Autodesk Inventor part; units mm, degrees
note: some values were not read from the file. Chosen so that the rebuilt part matches the saved one: direction of "Hole2".
(part 12 of 20)
  line L725 (-87.264021, -27.045907) -> (-87.291941, -27.048237)
  line L726 (-87.250271, -24.95924) -> (-87.458208, -24.976595)
  line L727 (-87.288621, -27.057017) -> (-87.239208, -27.052892)
  ellipse E573 centre (-87.05098, -26.778416) end of major axis (-86.983232, -26.537771) minor radius 0.214215 (-87.262006, -26.740129) -> (-87.262743, -26.851991) ccw
  ellipse E574 centre (-87.040523, -25.191443) end of major axis (-86.972774, -24.950798) minor radius 0.214215 (-87.251549, -25.153156) -> (-87.252286, -25.265018) ccw
  spline S72 degree 3 poles (-86.844242, -26.766257) (-86.846137, -26.752647) (-86.849873, -26.725818) (-86.862228, -26.68763) (-86.878945, -26.652628) (-86.900084, -26.621606) (-86.92513, -26.595311) (-86.953734, -26.574537) (-86.980247, -26.56254) (-87.002525, -26.556638) (-87.019846, -26.554098) (-87.037692, -26.553557) (-87.056005, -26.555112) (-87.074575, -26.558831) (-87.093006, -26.564642) (-87.110888, -26.572422) (-87.133717, -26.5852) (-87.16009, -26.605396) (-87.187412, -26.63502) (-87.209849, -26.669164) (-87.227399, -26.706727) (-87.23392, -26.733619) (-87.237193, -26.747114) knots 0 0 0 0 0.06705351 0.13217076 0.19521445 0.25608707 0.314845 0.37183317 0.42783149 0.45589727 0.48426542 0.51319288 0.54296576 0.57389196 0.60556318 0.63723227 0.66902668 0.73324746 0.79861392 0.865047 0.93227307 1 1 1 1
  spline S73 degree 3 poles (-87.262006, -26.740129) (-87.260244, -26.733331) (-87.256712, -26.719711) (-87.246016, -26.693462) (-87.227942, -26.662404) (-87.199749, -26.629194) (-87.166328, -26.600489) (-87.128819, -26.577002) (-87.088383, -26.559452) (-87.046165, -26.548593) (-87.010271, -26.545789) (-86.981977, -26.547757) (-86.961175, -26.551403) (-86.941138, -26.55724) (-86.922223, -26.565108) (-86.90469, -26.574815) (-86.883243, -26.589954) (-86.859658, -26.612961) (-86.836903, -26.6456) (-86.819582, -26.682128) (-86.807069, -26.721446) (-86.802924, -26.748832) (-86.800834, -26.762634) knots 0 0 0 0 0.03133748 0.06278121 0.12629735 0.19093644 0.25645898 0.32231967 0.3878749 0.45257734 0.51618281 0.54767829 0.57907039 0.61032535 0.64070557 0.67038635 0.69964994 0.75776174 0.81647804 0.87644136 0.93772561 1 1 1 1
  spline S74 degree 3 poles (-86.801575, -26.874947) (-86.803934, -26.887405) (-86.808531, -26.911671) (-86.823414, -26.945046) (-86.84347, -26.974042) (-86.868727, -26.998205) (-86.898529, -27.017194) (-86.932394, -27.030679) (-86.969811, -27.038356) (-87.010303, -27.03992) (-87.052914, -27.035123) (-87.095691, -27.024267) (-87.136319, -27.007228) (-87.173004, -26.984845) (-87.204936, -26.957641) (-87.227026, -26.931239) (-87.241417, -26.90832) (-87.250446, -26.890314) (-87.257822, -26.871543) (-87.2611, -26.858518) (-87.262743, -26.851991) knots 0 0 0 0 0.06022667 0.11730293 0.17254203 0.22724068 0.28263107 0.33984452 0.39989686 0.46369518 0.53205848 0.6034638 0.67318901 0.7411164 0.8073508 0.87214279 0.90417982 0.93607992 0.96796844 1 1 1 1
  spline S75 degree 3 poles (-87.23793, -26.858977) (-87.237265, -26.862275) (-87.23594, -26.868848) (-87.233332, -26.878531) (-87.230299, -26.888022) (-87.225663, -26.900374) (-87.218799, -26.91531) (-87.20898, -26.932343) (-87.197734, -26.948418) (-87.185176, -26.963452) (-87.171525, -26.9775) (-87.161568, -26.98592) (-87.156591, -26.990129) knots 0 0 0 0 0.06406043 0.12763921 0.19082759 0.25370622 0.37876994 0.50330734 0.62760512 0.75181377 0.87596664 1 1 1 1
  spline S76 degree 3 poles (-86.94314, -27.035596) (-86.939586, -27.03406) (-86.932537, -27.031015) (-86.922574, -27.025353) (-86.913208, -27.018983) (-86.904463, -27.011852) (-86.896326, -27.004009) (-86.888792, -26.995478) (-86.881851, -26.986289) (-86.875498, -26.976469) (-86.869724, -26.966046) (-86.864521, -26.955048) (-86.859882, -26.9435) (-86.855799, -26.931431) (-86.852262, -26.918867) (-86.849276, -26.905834) (-86.846786, -26.892364) (-86.845588, -26.883204) (-86.844982, -26.87857) knots 0 0 0 0 0.05963345 0.11825449 0.17626219 0.23403402 0.29191894 0.35023204 0.40925111 0.46921525 0.53032509 0.59274441 0.65660269 0.7219981 0.78900076 0.85765603 0.92798753 1 1 1 1
  spline S77 degree 3 poles (-86.833785, -25.179284) (-86.83568, -25.165674) (-86.839416, -25.138845) (-86.851771, -25.100657) (-86.868488, -25.065655) (-86.889626, -25.034633) (-86.914673, -25.008338) (-86.943277, -24.987564) (-86.969789, -24.975567) (-86.992068, -24.969665) (-87.009388, -24.967125) (-87.027235, -24.966584) (-87.045548, -24.968139) (-87.064118, -24.971858) (-87.082548, -24.977669) (-87.10043, -24.985449) (-87.12326, -24.998227) (-87.149633, -25.018423) (-87.176955, -25.048047) (-87.199392, -25.082191) (-87.216942, -25.119754) (-87.223463, -25.146646) (-87.226736, -25.160141) knots 0 0 0 0 0.06705351 0.13217076 0.19521445 0.25608707 0.314845 0.37183317 0.42783149 0.45589727 0.48426542 0.51319288 0.54296576 0.57389196 0.60556318 0.63723227 0.66902668 0.73324746 0.79861392 0.865047 0.93227307 1 1 1 1
  spline S78 degree 3 poles (-87.251549, -25.153156) (-87.249786, -25.146357) (-87.246255, -25.132738) (-87.235559, -25.106489) (-87.217485, -25.075431) (-87.189292, -25.042221) (-87.155871, -25.013516) (-87.118362, -24.990029) (-87.077926, -24.972479) (-87.035708, -24.96162) (-86.999814, -24.958816) (-86.97152, -24.960784) (-86.950718, -24.96443) (-86.930681, -24.970267) (-86.911765, -24.978135) (-86.894233, -24.987842) (-86.872786, -25.002981) (-86.849201, -25.025988) (-86.826446, -25.058627) (-86.809125, -25.095155) (-86.796612, -25.134473) (-86.792467, -25.161859) (-86.790377, -25.175661) knots 0 0 0 0 0.03133748 0.06278121 0.12629735 0.19093644 0.25645898 0.32231967 0.3878749 0.45257734 0.51618281 0.54767829 0.57907039 0.61032535 0.64070557 0.67038635 0.69964994 0.75776174 0.81647804 0.87644136 0.93772561 1 1 1 1
  spline S79 degree 3 poles (-86.791117, -25.287974) (-86.793477, -25.300432) (-86.798074, -25.324698) (-86.812957, -25.358073) (-86.833013, -25.387069) (-86.85827, -25.411232) (-86.888072, -25.430221) (-86.921937, -25.443706) (-86.959354, -25.451383) (-86.999846, -25.452947) (-87.042457, -25.44815) (-87.085233, -25.437294) (-87.125862, -25.420255) (-87.162546, -25.397872) (-87.194479, -25.370668) (-87.216569, -25.344266) (-87.23096, -25.321347) (-87.239988, -25.303341) (-87.247365, -25.28457) (-87.250643, -25.271545) (-87.252286, -25.265018) knots 0 0 0 0 0.06022667 0.11730293 0.17254203 0.22724068 0.28263107 0.33984452 0.39989686 0.46369518 0.53205848 0.6034638 0.67318901 0.7411164 0.8073508 0.87214279 0.90417982 0.93607992 0.96796844 1 1 1 1
  spline S80 degree 3 poles (-87.227473, -25.272004) (-87.226808, -25.275302) (-87.225483, -25.281875) (-87.222875, -25.291558) (-87.219842, -25.301049) (-87.215205, -25.3134) (-87.208342, -25.328337) (-87.198522, -25.34537) (-87.187277, -25.361445) (-87.174719, -25.376479) (-87.161068, -25.390527) (-87.151111, -25.398947) (-87.146134, -25.403156) knots 0 0 0 0 0.06406043 0.12763921 0.19082759 0.25370622 0.37876994 0.50330734 0.62760512 0.75181377 0.87596664 1 1 1 1
  spline S81 degree 3 poles (-86.932683, -25.448623) (-86.929129, -25.447087) (-86.92208, -25.444042) (-86.912117, -25.43838) (-86.90275, -25.43201) (-86.894006, -25.424879) (-86.885869, -25.417036) (-86.878334, -25.408505) (-86.871394, -25.399316) (-86.865041, -25.389496) (-86.859267, -25.379073) (-86.854064, -25.368074) (-86.849424, -25.356527) (-86.845342, -25.344458) (-86.841805, -25.331894) (-86.838819, -25.318861) (-86.836329, -25.305391) (-86.835131, -25.296231) (-86.834525, -25.291597) knots 0 0 0 0 0.05963345 0.11825449 0.17626219 0.23403402 0.29191894 0.35023204 0.40925111 0.46921525 0.53032509 0.59274441 0.65660269 0.7219981 0.78900076 0.85765603 0.92798753 1 1 1 1
  ellipse E575 centre (-86.922017, -26.784779) end of major axis (-86.901223, -27.033912) minor radius 0.122746 (-86.801575, -26.874947) -> (-86.800834, -26.762634) ccw
  ellipse E576 centre (-86.965424, -26.788402) end of major axis (-86.986218, -26.539268) minor radius 0.122746 (-86.844982, -26.87857) -> (-86.844242, -26.766257) ccw
  ellipse E577 centre (-86.91156, -25.197806) end of major axis (-86.890766, -25.446939) minor radius 0.122746 (-86.791117, -25.287974) -> (-86.790377, -25.175661) ccw
  ellipse E578 centre (-86.954967, -25.201429) end of major axis (-86.975761, -24.952295) minor radius 0.122746 (-86.834525, -25.291597) -> (-86.833785, -25.179284) ccw
  ellipse E579 centre (-87.026167, -26.785401) end of major axis (-87.093915, -27.026047) minor radius 0.214215 (-87.237193, -26.747114) -> (-87.23793, -26.858977) ccw
  ellipse E580 centre (-87.01571, -25.198428) end of major axis (-87.083458, -25.439074) minor radius 0.214215 (-87.226736, -25.160141) -> (-87.227473, -25.272004) ccw
  ellipse E581 centre (-87.096286, -27.093129) end of major axis (-86.808292, -27.095027) minor radius 0.045287 (-86.846258, -27.072261) -> (-87.239208, -27.052892) ccw
  ellipse E582 centre (-87.096286, -27.093129) end of major axis (-87.434279, -27.090902) minor radius 0.05315 (-86.802851, -27.068638) -> (-87.264021, -27.045907) ccw
  ellipse E583 centre (-87.082536, -25.006462) end of major axis (-87.420529, -25.004235) minor radius 0.05315 (-86.789101, -24.981971) -> (-87.250271, -24.95924) ccw
  line L728 (-86.643643, -27.113459) -> (-86.802851, -27.068638)
  line L729 (-86.789101, -24.981971) -> (-86.772465, -24.986654)
  line L730 (-86.756765, -24.991074) -> (-86.743873, -24.994703)
  line L731 (-86.685676, -27.117469) -> (-86.846258, -27.072261)
  line L732 (-107.562177, -25.014438) -> (-107.45568, -25.019413)
  ellipse E584 centre (-86.54231, -24.68723) end of major axis (-86.626787, -24.985498) minor radius 0.255849 (-86.550009, -24.992758) -> (-86.536151, -24.991163) ccw
  line L733 (-86.536151, -24.991163) -> (-86.46886, -25.010221)
  line L734 (-86.599622, -24.996924) -> (-86.550009, -24.992758)
  arc A8 (-108.822768, -25.15652) -> (-108.721613, -25.266481) centre (-108.550766, -25.007808) ccw
  ellipse E585 centre (-86.547255, -25.103114) end of major axis (-86.105319, -25.125457) minor radius 0.079087 (-86.348028, -25.04218) -> (-86.360093, -25.040539) ccw
  arc A9 (-85.268509, -25.261265) -> (-85.143186, -25.138916) centre (-85.413584, -24.987307) ccw
  ellipse E586 centre (-107.271615, -24.666993) end of major axis (-107.176326, -24.961985) minor radius 0.274042 (-107.284377, -24.971637) -> (-107.269597, -24.97313) ccw
  line L735 (-107.299761, -24.976606) -> (-107.284377, -24.971637)
  line L736 (-107.269597, -24.97313) -> (-107.130091, -24.98313)
  ellipse E587 centre (-87.344737, -24.633834) end of major axis (-87.318953, -24.94276) minor radius 0.152204 (-87.355436, -24.937038) -> (-87.346755, -24.939971) ccw
  line L737 (-87.455183, -24.945363) -> (-87.355436, -24.937038)
  ellipse E588 centre (-86.781051, -24.661503) end of major axis (-86.865059, -24.959903) minor radius 0.265627 (-86.783068, -24.967639) -> (-86.768741, -24.96601) ccw
  line L738 (-86.768741, -24.96601) -> (-86.718934, -24.980032)
  line L739 (-86.834568, -24.971938) -> (-86.783068, -24.967639)
  line L740 (-87.346755, -24.939971) -> (-87.294003, -24.954822)
  ellipse E589 centre (-87.203964, -25.032925) end of major axis (-86.761473, -25.035841) minor radius 0.069582 (-86.983801, -24.97398) -> (-87.009912, -24.971636) ccw
  arc A10 (-107.361771, -27.097474) -> (-107.495936, -27.121179) centre (-107.376234, -27.407136) ccw
  line L741 (-107.495936, -27.121179) -> (-107.541681, -27.140328)
  line L742 (-107.035954, -27.112691) -> (-107.361771, -27.097474)
  arc A11 (-107.768298, -27.148427) -> (-107.783494, -27.154591) centre (-107.659411, -27.438674) ccw
  arc A12 (-107.648929, -27.128852) -> (-107.740372, -27.139433) centre (-107.659411, -27.438674) ccw
  line L743 (-107.783494, -27.154591) -> (-107.873673, -27.193979)
  line L744 (-107.524335, -27.133067) -> (-107.648929, -27.128852)
  arc A13 (-106.402931, -32.497897) -> (-106.400859, -32.497157) centre (-106.805429, -31.367412) ccw
  line L745 (-87.818851, -31.56199) -> (-87.720015, -32.505823)
  line L746 (-106.184231, -31.56199) -> (-106.283067, -32.505823)
  arc A14 (-87.602223, -32.497157) -> (-87.600151, -32.497897) centre (-87.197653, -31.367412) ccw
  arc A15 (-90.598492, -35.33817) -> (-90.48289, -35.312603) centre (-90.799519, -34.155129) ccw
  line L747 (-90.29603, -34.046814) -> (-90.28314, -34.105092)
  arc A16 (-103.520192, -35.312603) -> (-103.40459, -35.33817) centre (-103.203563, -34.155129) ccw
  line L748 (-103.707052, -34.046814) -> (-103.719942, -34.105092)
  arc A17 (-107.267726, -34.321251) -> (-106.77775, -34.355522) centre (-106.940784, -33.166648) ccw
  line L749 (-108.036328, -21.696665) -> (-108.026854, -21.884052)
  line L750 (-107.975177, -22.906217) -> (-107.96796, -23.048964)
  line L751 (-107.657328, -29.193171) -> (-107.540315, -31.507663)
  line L752 (-107.48592, -32.583586) -> (-107.451463, -33.265126)
  arc A18 (-104.353756, -35.223246) -> (-104.235408, -35.229466) centre (-104.231678, -34.029472) ccw
  line L753 (-103.716719, -34.043774) -> (-103.719942, -34.105092)
  line L754 (-104.706079, -33.243459) -> (-104.756348, -34.199934)
  line L755 (-91.493695, -33.096855) -> (-91.477416, -33.173659)
  arc A19 (-88.109461, -35.54276) -> (-87.810531, -35.509047) centre (-88.093417, -34.342867) ccw
  line L756 (-87.667, -33.528456) -> (-87.560911, -34.469138)
  line L757 (-88.69143, -33.635739) -> (-88.584423, -34.584568)
  arc A20 (-106.192551, -35.509047) -> (-105.893621, -35.54276) centre (-105.909665, -34.342867) ccw
  line L758 (-105.311652, -33.635739) -> (-105.418659, -34.584568)
  line L759 (-106.336082, -33.528456) -> (-106.442171, -34.469138)
  line L760 (-102.509387, -33.096855) -> (-102.525666, -33.173659)
  arc A21 (-89.767674, -35.229466) -> (-89.649326, -35.223246) centre (-89.771404, -34.029472) ccw
  line L761 (-89.297003, -33.243459) -> (-89.246734, -34.199934)
  line L762 (-90.286363, -34.043774) -> (-90.28314, -34.105092)
  arc A22 (-87.225332, -34.355522) -> (-86.735356, -34.321251) centre (-87.062298, -33.166648) ccw
  line L763 (-85.966754, -21.696665) -> (-85.976228, -21.884052)
  line L764 (-86.027905, -22.906217) -> (-86.033482, -23.016517)
  line L765 (-86.344197, -29.162376) -> (-86.462767, -31.507663)
  line L766 (-86.517162, -32.583586) -> (-86.551619, -33.265126)
  line L767 (-106.187707, -21.753853) -> (-106.187436, -21.794963)
  line L768 (-106.139211, -29.113475) -> (-106.135988, -29.602592)
  line L769 (-88.008683, -28.994618) -> (-87.858681, -30.530102)
  line L770 (-105.994399, -28.994618) -> (-106.144401, -30.530102)
  line L771 (-87.815376, -21.753853) -> (-87.815646, -21.794963)
  line L772 (-87.863801, -29.102841) -> (-87.867094, -29.602592)
  ellipse E590 centre (-107.19283, -15.992439) end of major axis (-108.892291, -16.03526) minor radius 0.28459 (-108.378765, -15.817576) -> (-108.892291, -16.03526) ccw
  line L773 (-108.888419, -16.188929) -> (-108.892291, -16.03526)
  ellipse E591 centre (-86.810252, -15.992439) end of major axis (-85.110791, -16.03526) minor radius 0.28459 (-85.110791, -16.03526) -> (-85.624317, -15.817576) ccw
  line L774 (-85.114663, -16.188929) -> (-85.110791, -16.03526)
  ellipse E592 centre (-107.715782, -17.837411) end of major axis (-109.413614, -17.923248) minor radius 0.303839 (-108.663788, -17.631425) -> (-109.413614, -17.923248) ccw
  line L775 (-109.406367, -18.066578) -> (-109.413614, -17.923248)
  ellipse E593 centre (-86.2873, -17.837411) end of major axis (-84.589468, -17.923248) minor radius 0.303839 (-84.589468, -17.923248) -> (-85.339294, -17.631425) ccw
  line L776 (-84.596715, -18.066578) -> (-84.589468, -17.923248)
  ellipse E594 centre (-89.901015, -14.920785) end of major axis (-88.209069, -14.755498) minor radius 0.097712 (-88.209069, -14.755498) -> (-88.726459, -14.735759) ccw
  line L777 (-88.184691, -15.005043) -> (-88.209069, -14.755498)
  ellipse E595 centre (-104.102067, -14.920785) end of major axis (-105.794013, -14.755498) minor radius 0.097712 (-105.276623, -14.735759) -> (-105.794013, -14.755498) ccw
  line L778 (-105.818391, -15.005043) -> (-105.794013, -14.755498)
  ellipse E596 centre (-107.115847, -19.047722) end of major axis (-105.616323, -19.009938) minor radius 0.251109 (-106.242723, -18.822124) -> (-106.866306, -18.793926) ccw
  ellipse E597 centre (-107.115847, -19.047722) end of major axis (-105.21645, -18.999863) minor radius 0.318071 (-106.234573, -18.744288) -> (-108.180062, -18.810245) ccw
  ellipse E598 centre (-107.18538, -16.288111) end of major axis (-109.084778, -16.33597) minor radius 0.318071 (-107.887293, -16.009653) -> (-109.084778, -16.33597) ccw
  line L779 (-109.050041, -17.714567) -> (-109.084778, -16.33597)
  ellipse E599 centre (-89.550588, -19.969597) end of major axis (-87.66092, -19.771717) minor radius 0.08119 (-87.819088, -19.82131) -> (-87.877602, -19.756773) ccw
  ellipse E600 centre (-89.841934, -17.187367) end of major axis (-87.952267, -16.989487) minor radius 0.08119 (-88.062989, -16.97389) -> (-88.463494, -16.987448) ccw
  line L780 (-87.66092, -19.771717) -> (-87.86609, -17.812439)
  ellipse E601 centre (-104.452494, -19.969597) end of major axis (-106.342162, -19.771717) minor radius 0.08119 (-106.12548, -19.756773) -> (-106.183994, -19.82131) ccw
  ellipse E602 centre (-104.161148, -17.187367) end of major axis (-106.050815, -16.989487) minor radius 0.08119 (-105.539588, -16.987448) -> (-105.940093, -16.97389) ccw
  line L781 (-106.342162, -19.771717) -> (-106.136992, -17.812439)
  ellipse E603 centre (-86.887235, -19.047722) end of major axis (-85.387711, -19.085505) minor radius 0.251109 (-87.136776, -18.793926) -> (-87.760359, -18.822124) ccw
  ellipse E604 centre (-86.887235, -19.047722) end of major axis (-84.987838, -19.095581) minor radius 0.318071 (-85.82302, -18.810245) -> (-87.768509, -18.744288) ccw
  ellipse E605 centre (-86.817702, -16.288111) end of major axis (-84.918305, -16.33597) minor radius 0.318071 (-84.918305, -16.33597) -> (-86.115789, -16.009653) ccw
  line L782 (-84.953041, -17.714567) -> (-84.918305, -16.33597)
  ellipse E606 centre (-107.561776, -20.883606) end of major axis (-109.059863, -20.959344) minor radius 0.268093 (-106.281023, -20.681668) -> (-108.752123, -21.104847) ccw
  ellipse E607 centre (-107.561776, -20.883606) end of major axis (-109.459353, -20.979541) minor radius 0.339584 (-106.268597, -20.571487) -> (-108.746952, -21.207144) ccw
  ellipse E608 centre (-107.700878, -18.132204) end of major axis (-109.598455, -18.22814) minor radius 0.339584 (-108.216239, -17.830199) -> (-109.598455, -18.22814) ccw
  line L783 (-109.459353, -20.979541) -> (-109.598455, -18.22814)
  ellipse E609 centre (-89.493947, -21.924428) end of major axis (-87.605916, -21.7115) minor radius 0.04047 (-87.905161, -21.767333) -> (-87.910255, -21.723732) ccw
  ellipse E610 centre (-89.807666, -19.142698) end of major axis (-87.919635, -18.929769) minor radius 0.04047 (-87.969068, -18.926181) -> (-88.235125, -18.942892) ccw
  line L784 (-87.605916, -21.7115) -> (-87.824872, -19.770026)
  ellipse E611 centre (-104.509135, -21.924428) end of major axis (-106.397166, -21.7115) minor radius 0.04047 (-106.092827, -21.723732) -> (-106.097921, -21.767333) ccw
  ellipse E612 centre (-104.195416, -19.142698) end of major axis (-106.083447, -18.929769) minor radius 0.04047 (-105.767957, -18.942892) -> (-106.034014, -18.926181) ccw
  line L785 (-106.397166, -21.7115) -> (-106.17821, -19.770026)
  ellipse E613 centre (-86.441306, -20.883606) end of major axis (-84.943219, -20.959344) minor radius 0.268093 (-85.250959, -21.104847) -> (-87.722059, -20.681668) ccw
  ellipse E614 centre (-86.441306, -20.883606) end of major axis (-84.54373, -20.979541) minor radius 0.339584 (-85.25613, -21.207144) -> (-87.734485, -20.571487) ccw
  ellipse E615 centre (-86.302204, -18.132204) end of major axis (-84.404627, -18.22814) minor radius 0.339584 (-84.404627, -18.22814) -> (-85.786843, -17.830199) ccw
  line L786 (-84.54373, -20.979541) -> (-84.404627, -18.22814)
  ellipse E616 centre (-106.732899, -17.173539) end of major axis (-105.232932, -17.163655) minor radius 0.235872 (-106.209263, -16.949137) -> (-106.226441, -16.948259) ccw
  ellipse E617 centre (-106.732899, -17.173539) end of major axis (-104.832941, -17.161019) minor radius 0.298772 (-106.202823, -16.883218) -> (-107.873135, -16.941875) ccw
  ellipse E618 centre (-106.75112, -14.408434) end of major axis (-108.651078, -14.420953) minor radius 0.298772 (-108.571129, -14.33437) -> (-108.651078, -14.420953) ccw
  line L787 (-108.64147, -15.879063) -> (-108.651078, -14.420953)
  ellipse E619 centre (-89.600107, -18.000997) end of major axis (-87.709109, -17.816265) minor radius 0.109208 (-87.859598, -17.874433) -> (-87.980135, -17.786664) ccw
  ellipse E620 centre (-89.871895, -15.21887) end of major axis (-87.980896, -15.034138) minor radius 0.109208 (-87.980896, -15.034138) -> (-88.69346, -15.018318) ccw
  line L788 (-87.709109, -17.816265) -> (-87.980896, -15.034138)
  ellipse E621 centre (-104.402975, -18.000997) end of major axis (-106.293973, -17.816265) minor radius 0.109208 (-106.022947, -17.786664) -> (-106.143484, -17.874433) ccw
  ellipse E622 centre (-104.131188, -15.21887) end of major axis (-106.022186, -15.034138) minor radius 0.109208 (-105.309622, -15.018318) -> (-106.022186, -15.034138) ccw
  line L789 (-106.293973, -17.816265) -> (-106.022186, -15.034138)
  ellipse E623 centre (-87.270183, -17.173539) end of major axis (-85.770215, -17.183423) minor radius 0.235872 (-87.776641, -16.948259) -> (-87.793819, -16.949137) ccw
  ellipse E624 centre (-87.270183, -17.173539) end of major axis (-85.370224, -17.186059) minor radius 0.298772 (-86.129947, -16.941875) -> (-87.800259, -16.883218) ccw
  ellipse E625 centre (-87.251962, -14.408434) end of major axis (-85.352004, -14.420953) minor radius 0.298772 (-85.352004, -14.420953) -> (-85.431953, -14.33437) ccw
  line L790 (-85.361612, -15.879063) -> (-85.352004, -14.420953)
  line L791 (-105.746276, -23.38541) -> (-105.729813, -23.485843)
  line L792 (-105.713438, -23.585748) -> (-104.518837, -30.873787)
  line L793 (-100.540552, -31.290018) -> (-99.681906, -29.082528)
  line L794 (-100.540634, -31.290046) -> (-100.540552, -31.290018)
  line L795 (-105.168163, -17.859877) -> (-105.548042, -21.490716)
  line L796 (-105.745774, -23.380609) -> (-105.746276, -23.38541)
  line L797 (-105.168245, -17.859905) -> (-105.244123, -18.585136)
  line L798 (-100.612517, -31.282525) -> (-100.540634, -31.290046)
  line L799 (-104.518837, -30.873787) -> (-104.096258, -30.918)
  line L800 (-102.437806, -31.091516) -> (-100.540552, -31.290018)
  ellipse E626 centre (-105.168328, -17.859932) end of major axis (-105.221189, -18.365174) minor radius 0.000079 (-105.168245, -17.859904) -> (-105.143846, -17.626612) ccw
  ellipse E627 centre (-105.168328, -17.859932) end of major axis (-105.274051, -18.870417) minor radius 0.000159 (-105.168162, -17.859876) -> (-105.119364, -17.393293) ccw
  ellipse E628 centre (-104.487386, -11.346448) end of major axis (-104.381663, -10.335964) minor radius 0.000159 (-104.438421, -10.879809) -> (-104.381663, -10.335964) ccw
  ellipse E629 centre (-104.487386, -11.346448) end of major axis (-104.434524, -10.841206) minor radius 0.000079 (-104.462903, -11.113129) -> (-104.434524, -10.841206) ccw
  line L801 (-104.381663, -10.335964) -> (-104.071263, -10.368439)
  line L802 (-105.143846, -17.626613) -> (-104.462903, -11.113129)
  line L803 (-105.119364, -17.393293) -> (-104.438421, -10.879809)
  line L804 (-104.381826, -10.336018) -> (-105.376912, -10.232131)
  line L805 (-105.429773, -10.737374) -> (-105.376912, -10.232131)
  line L806 (-105.429773, -10.737374) -> (-104.434687, -10.84126)
  line L807 (-104.381826, -10.336018) -> (-104.434687, -10.84126)
  line L808 (-105.376912, -10.232131) -> (-105.377, -10.232161)
  line L809 (-104.434687, -10.84126) -> (-104.434524, -10.841206)
  line L810 (-104.381663, -10.335964) -> (-104.381826, -10.336018)
  line L811 (-101.001541, -16.931336) -> (-101.001541, -17.607529)
  line L812 (-93.001541, -16.931336) -> (-93.001541, -17.607529)
  line L813 (-101.001541, -16.931336) -> (-101.001541, -16.476694)
  line L814 (-93.001541, -16.931336) -> (-93.001541, -16.476694)
  line L815 (-101.001541, -16.476694) -> (-101.001541, -16.004474)
  line L816 (-93.001541, -16.004474) -> (-93.001541, -16.476694)
  line L817 (-92.680036, -10.077548) -> (-93.001541, -9.971815)
  line L818 (-93.001541, -10.477057) -> (-92.742184, -10.56235)
  line L819 (-101.001541, -9.971815) -> (-101.323047, -10.077548)
  line L820 (-101.260898, -10.56235) -> (-101.001541, -10.477057)
  line L821 (-93.46253, -31.290018) -> (-93.462448, -31.290046)
  line L822 (-94.321176, -29.082528) -> (-93.46253, -31.290018)
  line L823 (-89.484246, -30.873787) -> (-88.289644, -23.585748)
  line L824 (-88.273269, -23.485843) -> (-88.256806, -23.38541)
  line L825 (-88.758959, -18.585136) -> (-88.834837, -17.859905)
  line L826 (-88.83492, -17.859877) -> (-88.45504, -21.490716)
  line L827 (-88.257308, -23.380609) -> (-88.256806, -23.38541)
  line L828 (-93.462448, -31.290046) -> (-93.390565, -31.282525)
  line L829 (-93.46253, -31.290018) -> (-91.565276, -31.091516)
  line L830 (-89.906824, -30.918) -> (-89.484246, -30.873787)
  ellipse E630 centre (-88.834754, -17.859932) end of major axis (-88.887615, -17.35469) minor radius 0.000079 (-88.859236, -17.626613) -> (-88.834837, -17.859905) ccw
  ellipse E631 centre (-88.834754, -17.859932) end of major axis (-88.729031, -18.870417) minor radius 0.000159 (-88.883718, -17.393293) -> (-88.83492, -17.859876) ccw
  ellipse E632 centre (-89.515697, -11.346448) end of major axis (-89.621419, -10.335964) minor radius 0.000159 (-89.621419, -10.335964) -> (-89.564661, -10.879809) ccw
  ellipse E633 centre (-89.515697, -11.346448) end of major axis (-89.568558, -10.841206) minor radius 0.000079 (-89.568558, -10.841206) -> (-89.540179, -11.113129) ccw
  line L831 (-89.931819, -10.368439) -> (-89.621419, -10.335964)
  line L832 (-88.859236, -17.626613) -> (-89.540179, -11.113129)
  line L833 (-89.564661, -10.879809) -> (-88.883718, -17.393293)
  line L834 (-88.62617, -10.232131) -> (-89.621256, -10.336018)
  line L835 (-89.568395, -10.84126) -> (-89.621256, -10.336018)
  line L836 (-89.568395, -10.84126) -> (-88.573309, -10.737374)
  line L837 (-88.573309, -10.737374) -> (-88.62617, -10.232131)
  line L838 (-88.626082, -10.232161) -> (-88.62617, -10.232131)
  line L839 (-89.621256, -10.336018) -> (-89.621419, -10.335964)
  line L840 (-89.568558, -10.841206) -> (-89.568395, -10.84126)
  line L841 (-99.983458, -29.857787) -> (-99.001541, -33.451603)
  line L842 (-95.001541, -33.451603) -> (-94.019624, -29.857787)
  line L843 (-99.001541, -33.451603) -> (-95.001541, -33.451603)
  line L844 (-99.376982, -33.130004) -> (-99.001541, -34.494843)
  line L845 (-95.001541, -34.494843) -> (-94.628676, -33.139367)
  line L846 (-99.001541, -34.494843) -> (-95.001541, -34.494843)
  line L847 (-105.368984, -32.762749) -> (-106.506005, -25.260111)
  line L848 (-105.368932, -32.762729) -> (-105.368984, -32.762749)
  line L849 (-106.505954, -25.260091) -> (-105.368932, -32.762729)
  line L850 (-106.506005, -25.260111) -> (-106.505954, -25.260091)
  line L851 (-101.395958, -33.226918) -> (-100.612503, -31.28249)
  line L852 (-101.396009, -33.226938) -> (-101.395958, -33.226918)
  line L853 (-105.861231, -19.741934) -> (-106.505954, -25.260091)
  line L854 (-105.861282, -19.741953) -> (-106.506005, -25.260111)
  line L855 (-105.368984, -32.762749) -> (-101.396009, -33.226938)
  line L856 (-105.368932, -32.762729) -> (-101.395958, -33.226918)
  ellipse E634 centre (-105.861334, -19.741973) end of major axis (-105.920286, -20.246541) minor radius 0.000049 (-105.861282, -19.741952) -> (-105.834067, -19.508971) ccw
  ellipse E635 centre (-105.861334, -19.741973) end of major axis (-105.979238, -20.751109) minor radius 0.000097 (-105.861231, -19.741931) -> (-105.8068, -19.275969) ccw
  ellipse E636 centre (-105.101659, -13.237131) end of major axis (-104.983755, -12.227996) minor radius 0.000097 (-105.047126, -12.771129) -> (-104.983755, -12.227996) ccw
  ellipse E637 centre (-105.101659, -13.237131) end of major axis (-105.042707, -12.732563) minor radius 0.000049 (-105.074393, -13.00413) -> (-105.042707, -12.732563) ccw
  line L857 (-104.983755, -12.227996) -> (-104.584334, -12.274663)
  line L858 (-105.834067, -19.508972) -> (-105.074393, -13.00413)
  line L859 (-105.806801, -19.275971) -> (-105.047126, -12.771129)
  line L860 (-104.983856, -12.228035) -> (-105.97742, -12.11211)
  line L861 (-106.036372, -12.616678) -> (-105.97742, -12.11211)
  line L862 (-106.036372, -12.616678) -> (-105.042808, -12.732602)
  line L863 (-104.983856, -12.228035) -> (-105.042808, -12.732602)
  line L864 (-105.97742, -12.11211) -> (-105.97749, -12.112138)
  line L865 (-105.042808, -12.732602) -> (-105.042707, -12.732563)
  line L866 (-104.983755, -12.227996) -> (-104.983856, -12.228035)
  line L867 (-99.001541, -31.555877) -> (-101.001541, -24.285223)
  line L868 (-99.001541, -31.496991) -> (-99.001541, -31.555877)
  line L869 (-101.001541, -24.226337) -> (-99.001541, -31.496991)
  line L870 (-101.001541, -24.285223) -> (-101.001541, -24.226337)
  line L871 (-93.001541, -24.285223) -> (-95.001541, -31.555877)
  line L872 (-93.001541, -24.226337) -> (-93.001541, -24.285223)
  line L873 (-95.001541, -31.496991) -> (-93.001541, -24.226337)
  line L874 (-95.001541, -31.555877) -> (-95.001541, -31.496991)
  line L875 (-101.001541, -18.708096) -> (-101.001541, -24.226337)
  line L876 (-93.001541, -18.708096) -> (-93.001541, -24.226337)
  line L877 (-99.001541, -31.555877) -> (-95.001541, -31.555877)
  line L878 (-99.001541, -31.496991) -> (-95.001541, -31.496991)
  line L879 (-101.001541, -18.708096) -> (-101.001541, -18.255429)
  line L880 (-93.001541, -18.708096) -> (-93.001541, -18.255429)
  line L881 (-101.001541, -18.255429) -> (-101.001541, -17.607529)
  line L882 (-93.001541, -17.607529) -> (-93.001541, -18.255429)
  line L883 (-92.788959, -11.900633) -> (-93.001541, -11.822764)
  line L884 (-93.001541, -12.327339) -> (-92.848943, -12.383236)
  line L885 (-101.001541, -11.822764) -> (-101.214123, -11.900633)
  line L886 (-101.154139, -12.383236) -> (-101.001541, -12.327339)
  line L887 (-92.607124, -33.226918) -> (-92.607073, -33.226938)
  line L888 (-93.390579, -31.28249) -> (-92.607124, -33.226918)
  line L889 (-87.497077, -25.260111) -> (-88.634098, -32.762749)
  line L890 (-87.497128, -25.260091) -> (-87.497077, -25.260111)
  line L891 (-88.63415, -32.762729) -> (-87.497128, -25.260091)
  line L892 (-88.634098, -32.762749) -> (-88.63415, -32.762729)
  line L893 (-87.497077, -25.260111) -> (-88.1418, -19.741953)
  line L894 (-88.141851, -19.741934) -> (-87.497128, -25.260091)
  line L895 (-92.607073, -33.226938) -> (-88.634098, -32.762749)
  line L896 (-92.607124, -33.226918) -> (-88.63415, -32.762729)
  ellipse E638 centre (-88.141748, -19.741973) end of major axis (-88.2007, -19.237405) minor radius 0.000049 (-88.169015, -19.508972) -> (-88.1418, -19.741953) ccw
  ellipse E639 centre (-88.141748, -19.741973) end of major axis (-88.023844, -20.751109) minor radius 0.000097 (-88.196282, -19.275969) -> (-88.141851, -19.741931) ccw
  ellipse E640 centre (-88.901423, -13.237131) end of major axis (-89.019327, -12.227996) minor radius 0.000097 (-89.019327, -12.227996) -> (-88.955956, -12.771129) ccw
  ellipse E641 centre (-88.901423, -13.237131) end of major axis (-88.960375, -12.732563) minor radius 0.000049 (-88.960375, -12.732563) -> (-88.928689, -13.00413) ccw
  line L897 (-89.418748, -12.274663) -> (-89.019327, -12.227996)
  line L898 (-88.169015, -19.508972) -> (-88.928689, -13.00413)
  line L899 (-88.955956, -12.771129) -> (-88.196281, -19.275971)
  line L900 (-88.025663, -12.11211) -> (-89.019226, -12.228035)
  line L901 (-88.960274, -12.732602) -> (-89.019226, -12.228035)
  line L902 (-88.960274, -12.732602) -> (-87.966711, -12.616678)
  line L903 (-87.966711, -12.616678) -> (-88.025663, -12.11211)
  line L904 (-88.025592, -12.112138) -> (-88.025663, -12.11211)
  line L905 (-89.019226, -12.228035) -> (-89.019327, -12.227996)
  line L906 (-88.960375, -12.732563) -> (-88.960274, -12.732602)
  line L907 (-104.600226, -15.951564) -> (-104.781217, -17.861033)
  line L908 (-104.600262, -15.951566) -> (-104.669273, -16.679632)
  ellipse E642 centre (-104.600299, -15.951568) end of major axis (-104.648235, -16.457302) minor radius 0.000036 (-104.600262, -15.951564) -> (-104.578132, -15.718043) ccw
  ellipse E643 centre (-104.600299, -15.951568) end of major axis (-104.696172, -16.963035) minor radius 0.000072 (-104.600226, -15.95156) -> (-104.555965, -15.484517) ccw
  ellipse E644 centre (-103.982538, -9.431584) end of major axis (-103.886665, -8.420117) minor radius 0.000072 (-103.938204, -8.964537) -> (-103.886665, -8.420117) ccw
  ellipse E645 centre (-103.982538, -9.431584) end of major axis (-103.934601, -8.925851) minor radius 0.000036 (-103.960371, -9.19806) -> (-103.934601, -8.925851) ccw
  line L909 (-103.886665, -8.420117) -> (-101.606483, -8.636247)
  line L910 (-104.578132, -15.718045) -> (-103.960371, -9.19806)
  line L911 (-104.555965, -15.484521) -> (-103.938204, -8.964537)
  line L912 (-103.886736, -8.420122) -> (-104.8825, -8.325773)
  line L913 (-104.930437, -8.831506) -> (-104.8825, -8.325773)
  line L914 (-104.930437, -8.831506) -> (-103.934673, -8.925855)
  line L915 (-103.886736, -8.420122) -> (-103.934673, -8.925855)
  line L916 (-104.8825, -8.325773) -> (-104.882613, -8.32578)
  line L917 (-103.934673, -8.925855) -> (-103.934601, -8.925851)
  line L918 (-103.886665, -8.420117) -> (-103.886736, -8.420122)
  line L919 (-101.001541, -15.109953) -> (-101.001541, -16.004474)
  line L920 (-93.001541, -15.109953) -> (-93.001541, -16.004474)
  line L921 (-101.001541, -15.109953) -> (-101.001541, -14.653737)
  line L922 (-93.001541, -15.109953) -> (-93.001541, -14.653737)
  line L923 (-93.001541, -8.455297) -> (-93.001541, -7.991347)
  line L924 (-101.001541, -7.991347) -> (-101.001541, -8.455297)
  line L925 (-101.001541, -7.991347) -> (-93.001541, -7.991347)
  line L926 (-101.001541, -14.653737) -> (-101.001541, -8.455297)
  line L927 (-93.001541, -8.455297) -> (-93.001541, -14.653737)
  line L928 (-92.001541, -8.388269) -> (-93.001541, -8.090202)
  line L929 (-93.001541, -8.595937) -> (-92.524749, -8.738053)
  line L930 (-92.001541, -8.598801) -> (-92.001541, -8.388269)
  line L931 (-101.001541, -8.090202) -> (-102.001541, -8.388269)
  line L932 (-102.001541, -8.598801) -> (-102.001541, -8.388269)
  line L933 (-101.478333, -8.738053) -> (-101.001541, -8.595937)
  line L934 (-89.333809, -16.679632) -> (-89.40282, -15.951566)
  line L935 (-89.402856, -15.951564) -> (-89.221865, -17.861033)
  ellipse E646 centre (-89.402783, -15.951568) end of major axis (-89.45072, -15.445835) minor radius 0.000036 (-89.42495, -15.718045) -> (-89.40282, -15.951566) ccw
  ellipse E647 centre (-89.402783, -15.951568) end of major axis (-89.30691, -16.963035) minor radius 0.000072 (-89.447117, -15.484517) -> (-89.402856, -15.95156) ccw
  ellipse E648 centre (-90.020545, -9.431584) end of major axis (-90.116418, -8.420117) minor radius 0.000072 (-90.116418, -8.420117) -> (-90.064878, -8.964537) ccw
  ellipse E649 centre (-90.020545, -9.431584) end of major axis (-90.068481, -8.925851) minor radius 0.000036 (-90.068481, -8.925851) -> (-90.042711, -9.19806) ccw
  line L936 (-92.396599, -8.636247) -> (-90.116418, -8.420117)
  line L937 (-89.42495, -15.718045) -> (-90.042711, -9.19806)
  line L938 (-90.064878, -8.964537) -> (-89.447117, -15.484521)
  line L939 (-89.120582, -8.325773) -> (-90.116346, -8.420122)
  line L940 (-90.068409, -8.925855) -> (-90.116346, -8.420122)
  line L941 (-90.068409, -8.925855) -> (-89.072645, -8.831506)
  line L942 (-89.072645, -8.831506) -> (-89.120582, -8.325773)
  line L943 (-89.120469, -8.32578) -> (-89.120582, -8.325773)
  line L944 (-90.116346, -8.420122) -> (-90.116418, -8.420117)
  line L945 (-90.068481, -8.925851) -> (-90.068409, -8.925855)
  line L946 (-104.78319, -19.610031) -> (-104.762389, -19.411216)
  line L947 (-104.762161, -19.41114) -> (-104.782972, -19.610054)
  line L948 (-104.762389, -19.411216) -> (-104.762161, -19.41114)
  line L949 (-105.031615, -19.58404) -> (-105.031843, -19.584116)
  line L950 (-104.782972, -19.610054) -> (-105.031615, -19.58404)
  line L951 (-103.788401, -19.714112) -> (-103.767589, -19.515198)
  line L952 (-103.539758, -19.740127) -> (-103.788401, -19.714112)
  line L953 (-103.737696, -21.629888) -> (-103.986121, -21.603896)
  line L954 (-103.737468, -21.629812) -> (-103.737696, -21.629888)
  line L955 (-104.006922, -21.802712) -> (-103.986111, -21.603797)
  line L956 (-103.986111, -21.603797) -> (-103.737468, -21.629812)
  line L957 (-104.00715, -21.802788) -> (-104.006922, -21.802712)
  line L958 (-104.00715, -21.802788) -> (-104.271304, -21.77515)
  line L959 (-105.214334, -21.328345) -> (-105.031843, -19.584116)
  line L960 (-104.762161, -19.41114) -> (-103.767589, -19.515198)
  line L961 (-103.539758, -19.740127) -> (-103.737468, -21.629812)
  line L962 (-105.229325, -21.473725) -> (-105.031615, -19.58404)
  line L963 (-104.006922, -21.802712) -> (-105.001494, -21.698654)
  line L964 (-105.229325, -21.473725) -> (-104.980682, -21.49974)
  line L965 (-104.980682, -21.49974) -> (-105.001494, -21.698654)
  line L966 (-103.809212, -19.913026) -> (-103.965299, -21.404883)
  line L967 (-103.965299, -21.404883) -> (-104.95987, -21.300825)
  line L968 (-104.95987, -21.300825) -> (-104.803784, -19.808969)
  line L969 (-104.803784, -19.808969) -> (-103.809212, -19.913026)
  line L970 (-104.122484, -21.21122) -> (-104.003093, -20.070102)
  line L971 (-103.965299, -21.404883) -> (-104.122484, -21.21122)
  line L972 (-103.809212, -19.913026) -> (-104.003093, -20.070102)
  line L973 (-104.003093, -20.070102) -> (-104.646925, -20.002741)
  line L974 (-104.803784, -19.808969) -> (-104.646925, -20.002741)
  line L975 (-104.646925, -20.002741) -> (-104.766315, -21.143858)
  line L976 (-104.95987, -21.300825) -> (-104.766315, -21.143858)
  line L977 (-104.766315, -21.143858) -> (-104.122484, -21.21122)
  circle A23 centre (-104.35741, -20.346477) radius 0.1
  line L978 (-104.523452, -20.491903) -> (-104.489755, -20.169839)
  line L979 (-104.489788, -20.16985) -> (-104.489755, -20.169839)
  line L980 (-104.523484, -20.491914) -> (-104.489788, -20.16985)
  line L981 (-104.523484, -20.491914) -> (-104.523452, -20.491903)
  line L982 (-104.489755, -20.169839) -> (-104.191384, -20.201056)
  line L983 (-104.191384, -20.201056) -> (-104.22508, -20.523121)
  line L984 (-104.225113, -20.523132) -> (-104.22508, -20.523121)
  line L985 (-104.22508, -20.523121) -> (-104.523452, -20.491903)
  line L986 (-104.225113, -20.523132) -> (-104.523484, -20.491914)
  line L987 (-103.396493, -30.237119) -> (-103.595408, -30.216308)
  line L988 (-103.396265, -30.237043) -> (-103.396493, -30.237119)
  line L989 (-103.59518, -30.216232) -> (-103.396265, -30.237043)
  line L990 (-103.595408, -30.216308) -> (-103.59518, -30.216232)
  line L991 (-103.422508, -30.485762) -> (-103.396493, -30.237119)
  line L992 (-103.42228, -30.485686) -> (-103.422508, -30.485762)
  line L993 (-103.396265, -30.237043) -> (-103.42228, -30.485686)
  line L994 (-103.292425, -29.242449) -> (-103.266421, -28.993905)
  line L995 (-103.491122, -29.22166) -> (-103.49135, -29.221736)
  line L996 (-103.292208, -29.242472) -> (-103.491122, -29.22166)
  line L997 (-103.266193, -28.993829) -> (-103.292208, -29.242472)
  line L998 (-103.266421, -28.993905) -> (-103.266193, -28.993829)
  line L999 (-103.595408, -30.216308) -> (-103.49135, -29.221736)
  line L1000 (-101.532822, -30.683472) -> (-103.422508, -30.485762)
  line L1001 (-103.59518, -30.216232) -> (-103.491122, -29.22166)
  line L1002 (-103.266193, -28.993829) -> (-101.376508, -29.191539)
  line L1003 (-101.532594, -30.683396) -> (-103.42228, -30.485686)
  line L1004 (-101.203608, -29.460993) -> (-101.307666, -30.455565)
  line L1005 (-101.307894, -30.455641) -> (-101.50659, -30.434852)
  line L1006 (-101.532594, -30.683396) -> (-101.50658, -30.434753)
  line L1007 (-101.50658, -30.434753) -> (-101.307666, -30.455565)
  line L1008 (-101.307666, -30.455565) -> (-101.307894, -30.455641)
  line L1009 (-101.532822, -30.683472) -> (-101.532594, -30.683396)
  line L1010 (-101.203608, -29.460993) -> (-101.402522, -29.440182)
  line L1011 (-101.402522, -29.440182) -> (-101.376508, -29.191539)
  line L1012 (-103.093293, -29.263284) -> (-101.601436, -29.41937)
  line L1013 (-101.601436, -29.41937) -> (-101.705494, -30.413942)
  line L1014 (-101.705494, -30.413942) -> (-103.197351, -30.257855)
  line L1015 (-103.197351, -30.257855) -> (-103.093293, -29.263284)
  line L1016 (-101.795317, -29.576446) -> (-102.936435, -29.457056)
  line L1017 (-101.601436, -29.41937) -> (-101.795317, -29.576446)
  line L1018 (-103.093293, -29.263284) -> (-102.936435, -29.457056)
  line L1019 (-102.936435, -29.457056) -> (-103.003796, -30.100887)
  line L1020 (-103.197351, -30.257855) -> (-103.003796, -30.100887)
  line L1021 (-103.003796, -30.100887) -> (-101.862679, -30.220278)
  line L1022 (-101.705494, -30.413942) -> (-101.862679, -30.220278)
  line L1023 (-101.862679, -30.220278) -> (-101.795317, -29.576446)
  circle A24 centre (-102.660005, -29.811399) radius 0.1
  line L1024 (-102.51459, -29.977436) -> (-102.836655, -29.94374)
  line L1025 (-102.836687, -29.94375) -> (-102.836655, -29.94374)
  line L1026 (-102.514622, -29.977447) -> (-102.836687, -29.94375)
  line L1027 (-102.514622, -29.977447) -> (-102.51459, -29.977436)
  line L1028 (-102.836655, -29.94374) -> (-102.805437, -29.645368)
  line L1029 (-102.80547, -29.645379) -> (-102.805437, -29.645368)
  line L1030 (-102.836687, -29.94375) -> (-102.80547, -29.645379)
  line L1031 (-102.805437, -29.645368) -> (-102.483373, -29.679064)
  line L1032 (-102.483373, -29.679064) -> (-102.51459, -29.977436)
  line L1033 (-100.436541, -18.278179) -> (-100.436541, -18.477093)
  line L1034 (-100.436541, -18.477093) -> (-100.686541, -18.477093)
  line L1035 (-99.436541, -18.477093) -> (-99.436541, -18.278179)
  line L1036 (-99.186541, -18.477093) -> (-99.436541, -18.477093)
  line L1037 (-100.436541, -18.278179) -> (-99.436541, -18.278179)
  line L1038 (-99.186541, -18.477093) -> (-99.186541, -20.235039)
  line L1039 (-100.686541, -20.235039) -> (-100.686541, -18.477093)
  line L1040 (-99.436541, -18.676007) -> (-99.436541, -20.036387)
  line L1041 (-100.436541, -20.036387) -> (-100.436541, -18.676007)
  line L1042 (-100.436541, -18.676007) -> (-99.436541, -18.676007)
  line L1043 (-99.436541, -18.676007) -> (-99.596502, -18.929512)
  line L1044 (-100.436541, -18.676007) -> (-100.27658, -18.929512)
  ellipse E650 centre (-99.936541, -19.239499) end of major axis (-99.836541, -19.239499) minor radius 0.099457
  ellipse E651 centre (-99.936541, -19.244703) end of major axis (-99.836541, -19.244703) minor radius 0.099457 (-100.036541, -19.244703) -> (-99.836541, -19.244703) ccw
  line L1045 (-100.036541, -19.244703) -> (-100.036541, -19.239499)
  line L1046 (-99.836541, -19.244703) -> (-99.836541, -19.239499)
  line L1047 (-100.086541, -19.405735) -> (-100.086541, -19.083671)
  line L1048 (-100.086541, -19.416282) -> (-100.086541, -19.405735)
  line L1049 (-100.086541, -19.083671) -> (-99.786541, -19.083671)
  line L1050 (-99.786541, -19.083671) -> (-99.786541, -19.405735)
  line L1051 (-99.786541, -19.416282) -> (-99.786541, -19.405735)
  line L1052 (-99.786541, -19.405735) -> (-100.086541, -19.405735)
  line L1053 (-98.151541, -28.845483) -> (-97.951541, -28.845483)
  line L1054 (-98.151541, -28.92741) -> (-98.151541, -28.845483)
  line L1055 (-97.951541, -29.094126) -> (-97.951541, -29.175742)
  line L1056 (-97.951541, -28.845483) -> (-97.951541, -29.094126)
  line L1057 (-97.951541, -27.850913) -> (-98.151541, -27.850913)
  line L1058 (-97.951541, -27.602271) -> (-97.951541, -27.850913)
  line L1059 (-98.151541, -28.845483) -> (-98.151541, -27.850913)
  line L1060 (-97.951541, -27.602271) -> (-96.051541, -27.602271)
  line L1061 (-96.051541, -29.094126) -> (-97.951541, -29.094126)
  line L1062 (-95.851541, -27.850913) -> (-95.851541, -28.845483)
  line L1063 (-96.051541, -29.094126) -> (-96.051541, -28.845483)
  line L1064 (-96.051541, -28.845483) -> (-95.851541, -28.845483)
  line L1065 (-95.851541, -28.845483) -> (-95.851541, -28.92741)
  line L1066 (-96.051541, -29.175742) -> (-96.051541, -29.094126)
  line L1067 (-95.851541, -27.850913) -> (-96.051541, -27.850913)
  line L1068 (-96.051541, -27.850913) -> (-96.051541, -27.602271)
  line L1069 (-97.751541, -27.850913) -> (-96.251541, -27.850913)
  line L1070 (-96.251541, -27.850913) -> (-96.251541, -28.845483)
  line L1071 (-96.251541, -28.845483) -> (-97.751541, -28.845483)
  line L1072 (-97.751541, -28.845483) -> (-97.751541, -27.850913)
  line L1073 (-96.251541, -27.850913) -> (-96.392154, -28.073756)
  line L1074 (-97.751541, -27.850913) -> (-97.610928, -28.073756)
  line L1075 (-97.751541, -28.845483) -> (-97.612442, -28.789238)
  line L1076 (-96.251541, -28.845483) -> (-96.390641, -28.789238)
  ellipse E652 centre (-97.263452, -28.426252) end of major axis (-97.163452, -28.426252) minor radius 0.099457
  line L1077 (-97.363452, -28.430745) -> (-97.363452, -28.426252)
  line L1078 (-97.163452, -28.430745) -> (-97.163452, -28.426252)
  line L1079 (-92.496492, -30.434852) -> (-92.695188, -30.455641)
  line L1080 (-92.695416, -30.455565) -> (-92.496502, -30.434753)
  line L1081 (-92.695188, -30.455641) -> (-92.695416, -30.455565)
  line L1082 (-92.470488, -30.683396) -> (-92.47026, -30.683472)
  line L1083 (-92.496502, -30.434753) -> (-92.470488, -30.683396)
  line L1084 (-92.60056, -29.440182) -> (-92.799474, -29.460993)
  line L1085 (-92.626574, -29.191539) -> (-92.60056, -29.440182)
  line L1086 (-90.736661, -28.993905) -> (-90.710657, -29.242449)
  line L1087 (-90.736889, -28.993829) -> (-90.736661, -28.993905)
  line L1088 (-90.51196, -29.22166) -> (-90.710875, -29.242472)
  line L1089 (-90.710875, -29.242472) -> (-90.736889, -28.993829)
  line L1090 (-90.511732, -29.221736) -> (-90.51196, -29.22166)
  line L1091 (-90.511732, -29.221736) -> (-90.407674, -30.216308)
  line L1092 (-90.580574, -30.485762) -> (-92.47026, -30.683472)
  line L1093 (-92.695416, -30.455565) -> (-92.799474, -29.460993)
  line L1094 (-92.626574, -29.191539) -> (-90.736889, -28.993829)
  line L1095 (-90.580802, -30.485686) -> (-92.470488, -30.683396)
  line L1096 (-90.51196, -29.22166) -> (-90.407902, -30.216232)
  line L1097 (-90.407674, -30.216308) -> (-90.606589, -30.237119)
  line L1098 (-90.606589, -30.237119) -> (-90.580574, -30.485762)
  line L1099 (-90.580802, -30.485686) -> (-90.606817, -30.237043)
  line L1100 (-90.606817, -30.237043) -> (-90.407902, -30.216232)
  line L1101 (-90.407902, -30.216232) -> (-90.407674, -30.216308)
  line L1102 (-90.606817, -30.237043) -> (-90.606589, -30.237119)
  line L1103 (-90.580574, -30.485762) -> (-90.580802, -30.485686)
  line L1104 (-92.401646, -29.41937) -> (-90.909789, -29.263284)
  line L1105 (-90.909789, -29.263284) -> (-90.805731, -30.257855)
  line L1106 (-90.805731, -30.257855) -> (-92.297588, -30.413942)
  line L1107 (-92.297588, -30.413942) -> (-92.401646, -29.41937)
  line L1108 (-91.066647, -29.457056) -> (-92.207765, -29.576446)
  line L1109 (-90.909789, -29.263284) -> (-91.066647, -29.457056)
  line L1110 (-92.401646, -29.41937) -> (-92.207765, -29.576446)
  line L1111 (-92.207765, -29.576446) -> (-92.140403, -30.220278)
  line L1112 (-92.297588, -30.413942) -> (-92.140403, -30.220278)
  line L1113 (-92.140403, -30.220278) -> (-90.999286, -30.100887)
  line L1114 (-90.805731, -30.257855) -> (-90.999286, -30.100887)
  line L1115 (-90.999286, -30.100887) -> (-91.066647, -29.457056)
  circle A25 centre (-91.864056, -29.865907) radius 0.1
  line L1116 (-91.687406, -29.998247) -> (-92.009471, -30.031944)
  line L1117 (-92.009439, -30.031955) -> (-92.009471, -30.031944)
  line L1118 (-91.687374, -29.998258) -> (-92.009439, -30.031955)
  line L1119 (-91.687374, -29.998258) -> (-91.687406, -29.998247)
  line L1120 (-92.009471, -30.031944) -> (-92.040689, -29.733572)
  line L1121 (-92.040689, -29.733572) -> (-91.718624, -29.699876)
  line L1122 (-91.718591, -29.699887) -> (-91.718624, -29.699876)
  line L1123 (-91.718624, -29.699876) -> (-91.687406, -29.998247)
  line L1124 (-91.718591, -29.699887) -> (-91.687374, -29.998258)
  line L1125 (-98.151541, -32.701603) -> (-97.951541, -32.701603)
  line L1126 (-97.951541, -32.701603) -> (-97.951541, -32.951603)
  line L1127 (-97.951541, -31.701603) -> (-98.151541, -31.701603)
  line L1128 (-97.951541, -31.555877) -> (-97.951541, -31.701603)
  line L1129 (-98.151541, -32.701603) -> (-98.151541, -31.701603)
  line L1130 (-96.051541, -32.951603) -> (-97.951541, -32.951603)
  line L1131 (-95.851541, -31.701603) -> (-95.851541, -32.701603)
  line L1132 (-96.051541, -32.951603) -> (-96.051541, -32.701603)
  line L1133 (-96.051541, -32.701603) -> (-95.851541, -32.701603)
  line L1134 (-95.851541, -31.701603) -> (-96.051541, -31.701603)
  line L1135 (-96.051541, -31.701603) -> (-96.051541, -31.555877)
  line L1136 (-97.751541, -31.701603) -> (-96.251541, -31.701603)
  line L1137 (-96.251541, -31.701603) -> (-96.251541, -32.701603)
  line L1138 (-96.251541, -32.701603) -> (-97.751541, -32.701603)
  line L1139 (-97.751541, -32.701603) -> (-97.751541, -31.701603)
  line L1140 (-96.427868, -31.87793) -> (-97.575214, -31.87793)
  line L1141 (-96.251541, -31.701603) -> (-96.427868, -31.87793)
  line L1142 (-97.751541, -31.701603) -> (-97.575214, -31.87793)
  line L1143 (-97.575214, -31.87793) -> (-97.575214, -32.525276)